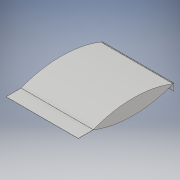
# Autodesk Inventor part: Futrterbeutel
Saved by Autodesk Inventor 2018 (Build 220112000, 112)
## iProperties
Created: 2018-03-14
Part Number: Futrterbeutel
Material: Generisch
Document SubType Name: Modeling
Designer: Julian
Density: 1 g/cm^3
Appearance: Vorgabe
Author: Julian
Autodesk Inventor part; units mm, degrees
ref_plane "YZ Plane" through (0, 0, 0) normal (1, 0, 0) x (0, 1, 0)
ref_plane "XZ Plane" through (0, 0, 0) normal (0, 1, 0) x (-1, 0, 0)
ref_plane "XY Plane" through (0, 0, 0) normal (0, 0, 1) x (1, 0, 0)
sketch "Skizze1" plane through (0, 0, 0) normal (1, 0, 0) x (0, 1, 0)
  line L0 (0, 0) -> (127.2, 0)
  line L1 (127.2, 0) -> (126, 0)
  line L2 (0, 0) -> (10, 0)
  line L3 (10, 0) -> (68, 0)
  line L4 (68, 0) -> (68, -10)
  line L5 (68, -10) -> (68, 10)
  line L6 (0, 0) -> (0, -0.1)
  line L7 (0, -0.1) -> (20, -0.1)
  line L8 (0, 0) -> (0, 0.1)
  line L9 (0, 0.1) -> (20, 0.1)
  line L10 (127.2, 0.1) -> (126, 0.1)
  line L11 (126, -0.1) -> (127, -0.1)
  line L12 (127, -0.1) -> (127, -9.1)
  line L13 (127, -9.1) -> (127.2, -9.1)
  line L14 (127.2, -9.1) -> (127.2, 0.1)
  arc A0 (20, -0.1) -> (126, -0.1) centre (73, 135.5561) ccw
  arc A1 (126, 0.1) -> (20, 0.1) centre (73, -135.5561) ccw
  dimension "d2" = 10
  dimension "d3" = 10
  dimension "d4" = 20
  dimension "d7" = 0.1
  dimension "d8" = 20
  dimension "d9" = 0.1
  dimension "d10" = 20
  dimension "d14" = 1
  dimension "d15" = 9
  dimension "d16" = 0.2
  dimension "d17" = 0.1
  dimension "d18" = 0.1
  constraints: 30 end point, 6 point on circle, 5 perpendicular, 5 point on line, 2 centre point, 2 horizontal, 2 vertical
  measures "d2" distance of L0.start L2.end
  measures "d3" distance of L3.end L4.end
  measures "d4" distance of L4.end L5.end
  measures "d7" distance of L0.start L6.end
  measures "d8" distance of L6.end L7.end
  measures "d9" distance of L0.start L8.end
  measures "d10" distance of L8.end L9.end
  measures "d14" distance of L11.start L11.end
  measures "d15" distance of L11.end L12.end
  measures "d16" distance of L12.end L13.end
  measures "d17" distance between parallel lines of L0 L10
  measures "d18" distance between parallel lines of L1 L11
extrude "Extrusion1" add sketch "Skizze1" along normal blind 96
